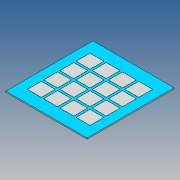
# Autodesk Inventor part: botonera
Saved by Autodesk Inventor 2017 (Build 210142000, 142)
## iProperties
Part Number: botonera
Material: Genérico
Document SubType Name: Modeling
Designer: Leo
Density: 1 g/cm^3
Appearance: Valor por defecto
Author: Leo
Autodesk Inventor part; units mm, degrees
ref_plane "YZ Plane" through (0, 0, 0) normal (1, 0, 0) x (0, 1, 0)
ref_plane "XZ Plane" through (0, 0, 0) normal (0, 1, 0) x (-1, 0, 0)
ref_plane "XY Plane" through (0, 0, 0) normal (0, 0, 1) x (1, 0, 0)
sketch "Boceto1" plane through (0, 0, 0) normal (0, 0, 1) x (1, 0, 0)
  line L0 (-35, 37.5) -> (35, 37.5)
  line L1 (35, 37.5) -> (35, -37.5)
  line L2 (35, -37.5) -> (-35, -37.5)
  line L3 (-35, -37.5) -> (-35, 37.5)
  point P0 (0, 0)
  point P1 (-35, 0)
  point P2 (0, 37.5)
  dimension "d0" = 70
  dimension "d1" = 75
  constraints: 8 end point, 2 midpoint, 2 parallel, 1 horizontal, 1 horizontal alignment, 1 perpendicular, 1 vertical alignment
  measures "d0" distance of L0.start L0.end
  measures "d1" distance of L2.end L0.start
extrude "Extrusión1" add sketch "Boceto1" along normal blind 1
sketch "Boceto2" plane through (0, 0, 1) normal (0, 0, 1) x (1, 0, 0)
  line L0 (-27, -27) -> (-15, -27)
  line L1 (-15, -27) -> (-15, -15)
  line L2 (-15, -15) -> (-27, -15)
  line L3 (-27, -15) -> (-27, -27)
  line L4 (-13, -27) -> (-1, -27)
  line L5 (-1, -27) -> (-1, -15)
  line L6 (-1, -15) -> (-13, -15)
  line L7 (-13, -15) -> (-13, -27)
  line L8 (1, -27) -> (13, -27)
  line L9 (13, -27) -> (13, -15)
  line L10 (13, -15) -> (1, -15)
  line L11 (1, -15) -> (1, -27)
  line L12 (15, -27) -> (27, -27)
  line L13 (27, -27) -> (27, -15)
  line L14 (27, -15) -> (15, -15)
  line L15 (15, -15) -> (15, -27)
  line L16 (-27, -13) -> (-15, -13)
  line L17 (-15, -13) -> (-15, -1)
  line L18 (-15, -1) -> (-27, -1)
  line L19 (-27, -1) -> (-27, -13)
  line L20 (-13, -13) -> (-1, -13)
  line L21 (-1, -13) -> (-1, -1)
  line L22 (-1, -1) -> (-13, -1)
  line L23 (-13, -1) -> (-13, -13)
  line L24 (1, -13) -> (13, -13)
  line L25 (13, -13) -> (13, -1)
  line L26 (13, -1) -> (1, -1)
  line L27 (1, -1) -> (1, -13)
  line L28 (15, -13) -> (27, -13)
  line L29 (27, -13) -> (27, -1)
  line L30 (27, -1) -> (15, -1)
  line L31 (15, -1) -> (15, -13)
  line L32 (-27, 1) -> (-15, 1)
  line L33 (-15, 1) -> (-15, 13)
  line L34 (-15, 13) -> (-27, 13)
  line L35 (-27, 13) -> (-27, 1)
  line L36 (-13, 1) -> (-1, 1)
  line L37 (-1, 1) -> (-1, 13)
  line L38 (-1, 13) -> (-13, 13)
  line L39 (-13, 13) -> (-13, 1)
  line L40 (1, 1) -> (13, 1)
  line L41 (13, 1) -> (13, 13)
  line L42 (13, 13) -> (1, 13)
  line L43 (1, 13) -> (1, 1)
  line L44 (15, 1) -> (27, 1)
  line L45 (27, 1) -> (27, 13)
  line L46 (27, 13) -> (15, 13)
  line L47 (15, 13) -> (15, 1)
  line L48 (-27, 15) -> (-15, 15)
  line L49 (-15, 15) -> (-15, 27)
  line L50 (-15, 27) -> (-27, 27)
  line L51 (-27, 27) -> (-27, 15)
  line L52 (-13, 15) -> (-1, 15)
  line L53 (-1, 15) -> (-1, 27)
  line L54 (-1, 27) -> (-13, 27)
  line L55 (-13, 27) -> (-13, 15)
  line L56 (1, 15) -> (13, 15)
  line L57 (13, 15) -> (13, 27)
  line L58 (13, 27) -> (1, 27)
  line L59 (1, 27) -> (1, 15)
  line L60 (15, 15) -> (27, 15)
  line L61 (27, 15) -> (27, 27)
  line L62 (27, 27) -> (15, 27)
  line L63 (15, 27) -> (15, 15)
  line L64 (-1, -1) -> (1, 1) construction
  point P0 (0, 0)
  point P1 (0, 0)
  dimension "d6" = 14
  dimension "d9" = 14
  dimension "d12" = 12
  constraints: 130 end point, 2 collinear, 2 horizontal, 2 parallel, 2 perpendicular, 1 coincident, 1 midpoint, 1 vertical, 118 other
  measures "d6" distance of L0.start L4.start
  measures "d9" distance of L0.start L16.start
  measures "d12" distance of L0.start L0.end
extrude "Extrusión2" add sketch "Boceto2" along normal blind 0.1
equation "\"d9\" = d6"
